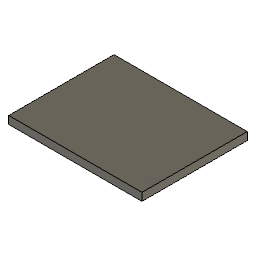
assembely (Autodesk Fusion 360 archive; units mm, degrees)
design "temp_sensor"
part number: 2025-12-15-20-50-01-731
Autodesk Fusion 360 part; units mm, degrees
sketch "Sketch1" plane through (0, 0, 0) normal (0, 0, 1) x (1, 0, 0)
  line L0 (0, 0) -> (25.3, 0)
  line L1 (25.3, 0) -> (25.3, 20)
  line L2 (25.3, 20) -> (0, 20)
  line L3 (0, 20) -> (0, 0)
  dimension "d1" = 25.3
  dimension "d2" = 20
  constraint horizontal L0
  constraint vertical L1
  constraint horizontal L2
  constraint vertical L3
  constraint coincident L0.start L3.end
  measures "d1" distance of L0.start L0.end
  measures "d2" distance of L0.start L2.end
extrude "Extrude1" add sketch "Sketch1" along normal blind 1.5

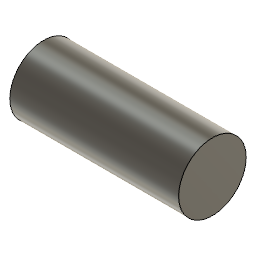
design "baterie"
part number: 2025-12-20-17-38-36-639
Autodesk Fusion 360 part; units mm, degrees
sketch "Sketch1" plane through (0, 0, 0) normal (1, 0, 0) x (0, 1, 0)
  circle A0 centre (0, 0) radius 13
  dimension "d1" = 26
  constraint coincident A0.centre origin
  measures "d1" diameter of A0
extrude "Extrude1" add sketch "Sketch1" along normal blind 65

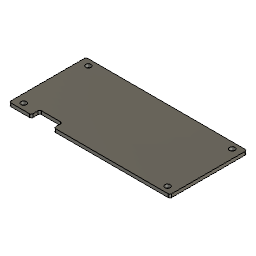
design "wood_back"
part number: 2025-12-15-21-34-38-126
Autodesk Fusion 360 part; units mm, degrees
sketch "Sketch1" plane through (0, 0, 0) normal (0, 0, 1) x (1, 0, 0)
  line L0 (0, 0) -> (96, 0)
  line L1 (96, 0) -> (96, 46)
  line L2 (96, 46) -> (0, 46)
  line L3 (0, 46) -> (0, 0)
  dimension "d1" = 96
  dimension "d2" = 46
  constraint horizontal L0
  constraint vertical L1
  constraint horizontal L2
  constraint vertical L3
  constraint coincident L0.start L3.end
  measures "d1" distance of L0.start L0.end
  measures "d2" distance of L0.start L2.end
extrude "Extrude1" add sketch "Sketch1" along normal blind 2
fillet "Fillet1" radius 1 4 edges at (96, 0, 1) (96, 46, 1) (0, 0, 1) (0, 46, 1)
sketch "Sketch2" plane through (0, 0, 2) normal (0, 0, 1) x (-1, 0, 0)
  arc A0 (-1, -46) -> (0, -45) centre (-1, -45) ccw
  line L0 (0, -45) -> (0, -1)
  arc A1 (0, -1) -> (-1, 0) centre (-1, -1) ccw
  line L1 (-1, 0) -> (-95, 0)
  arc A2 (-95, 0) -> (-96, -1) centre (-95, -1) ccw
  line L2 (-96, -1) -> (-96, -45)
  arc A3 (-96, -45) -> (-95, -46) centre (-95, -45) ccw
  line L3 (-95, -46) -> (-1, -46)
  line L4 (-13.3, 0) -> (-26.73, 0)
  line L5 (-26.73, 0) -> (-26.73, -4.065)
  line L6 (-25.73, -5.065) -> (-14.3, -5.065)
  line L7 (-13.3, -4.065) -> (-13.3, 0)
  arc A4 (-14.3, -5.065) -> (-13.3, -4.065) centre (-14.3, -4.065) ccw
  arc A5 (-26.73, -4.065) -> (-25.73, -5.065) centre (-25.73, -4.065) ccw
  point P0 (-13.3, -5.065)
  dimension "d7" = 13.43
  dimension "d8" = 5.065
  dimension "d9" = 13.3
  dimension "d10" = 5.065
  dimension "d11" = 1
  dimension "d12" = 1
  constraint horizontal L4
  constraint vertical L5
  constraint horizontal L6
  constraint vertical L7
  constraint coincident P0 L6
  constraint coincident P0 L7
  constraint tangent L6 A4
  constraint tangent L7 A4
  constraint tangent L5 A5
  constraint tangent L6 A5
  measures "d7" distance of L4.start L4.end
  measures "d8" distance of L4.start P0
  measures "d9" distance of L0 L7
  measures "d10" distance of L1 L6
  measures "d11" radius of A4
  measures "d12" radius of A5
extrude "Extrude2" cut sketch "Sketch2" against normal blind 2 contours L1 L4 L5 L6 L7 A4 A5
fillet "Fillet4" radius 1 2 edges at (13.3, 0, 1) (26.73, 0, 1)
sketch "Sketch5" plane through (0, 0, 2) normal (0, 0, 1) x (-1, 0, 0)
  arc A0 (-26.73, -1) -> (-27.73, 0) centre (-27.73, -1) ccw
  line L0 (-27.73, 0) -> (-95, 0)
  arc A1 (-95, 0) -> (-96, -1) centre (-95, -1) ccw
  line L1 (-96, -1) -> (-96, -45)
  arc A2 (-96, -45) -> (-95, -46) centre (-95, -45) ccw
  line L2 (-95, -46) -> (-1, -46)
  arc A3 (-1, -46) -> (0, -45) centre (-1, -45) ccw
  line L3 (0, -45) -> (0, -1)
  arc A4 (0, -1) -> (-1, 0) centre (-1, -1) ccw
  line L4 (-1, 0) -> (-12.3, 0)
  arc A5 (-12.3, 0) -> (-13.3, -1) centre (-12.3, -1) ccw
  line L5 (-13.3, -1) -> (-13.3, -4.065)
  arc A6 (-14.3, -5.065) -> (-13.3, -4.065) centre (-14.3, -4.065) ccw
  line L6 (-14.3, -5.065) -> (-25.73, -5.065)
  arc A7 (-26.73, -4.065) -> (-25.73, -5.065) centre (-25.73, -4.065) ccw
  line L7 (-26.73, -4.065) -> (-26.73, -1)
  circle A8 centre (-5.1, -3.75) radius 1.6
  circle A9 centre (-5.1, -42.25) radius 1.6
  circle A10 centre (-90.9, -3.75) radius 1.6
  circle A11 centre (-90.9, -42.25) radius 1.6
  dimension "d33" = 3.2
  dimension "d34" = 3.75
  dimension "d35" = 5.1
  dimension "d36" = 3.2
  dimension "d37" = 3.75
  dimension "d38" = 5.1
  dimension "d39" = 3.2
  dimension "d40" = 5.1
  dimension "d41" = 3.75
  dimension "d42" = 3.2
  dimension "d43" = 3.75
  dimension "d44" = 5.1
  measures "d33" diameter of A8
  measures "d34" distance of L4 A8.centre
  measures "d35" distance of L3 A8.centre
  measures "d36" diameter of A9
  measures "d37" distance of L2 A9.centre
  measures "d38" distance of L3 A9.centre
  measures "d39" diameter of A10
  measures "d40" distance of L1 A10.centre
  measures "d41" distance of L0 A10.centre
  measures "d42" diameter of A11
  measures "d43" distance of L2 A11.centre
  measures "d44" distance of L1 A11.centre
extrude "Extrude5" cut sketch "Sketch5" against normal blind 2 contours A8 | A9 | A10 | A11
equation "d8 = 4.69 mm - 0.375 mm + 0.75 mm"
equation "d10 = 4.69 mm - 0.375 mm + 0.75 mm"

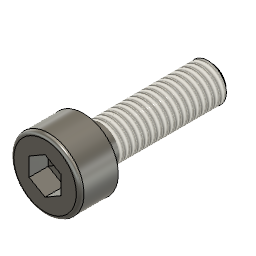
design "Broached Hexagon Socket Head Cap Screw ASME B18.3.1M - M3x0.5 x 10 Steel Grade 2 Plain"
description: Broached Hexagon Socket Head Cap Screw ASME B18.3.1M - M3x0.5 x 10
part number: BSHCS ASME B18.3.1M - M3x0.5 x 10 Steel Grade 2 Plain
Autodesk Fusion 360 part; units mm, degrees
sketch "Sketch1" plane through (0, 0, 0) normal (0, 1, 0) x (1, 0, 0)
  line L0 (-1.5, 0) -> (-1.5, 10)
  line L1 (-1.5, 10) -> (0, 10)
  line L2 (0, 10) -> (0, -3)
  line L3 (-1.5, 0) -> (-2.75, 0)
  line L4 (-2.75, 0) -> (-2.75, -3)
  line L5 (-2.75, -3) -> (0, -3)
  dimension "d101" = 10
  dimension "d102" = 3
  dimension "d109" = 5.5
  dimension "d110" = 3
  constraint perpendicular L0 L1
  constraint collinear origin L1.end L2.end
  constraint perpendicular L0 L3
  constraint coincident origin L3
  constraint vertical L2
  constraint coincident L2 L5.end
  constraint perpendicular L2 L5
  measures "d101" distance of origin L1
  measures "d102" distance of L3.end L5
revolve "Revolve1" add sketch "Sketch1" angle 360 about axis through (0, 0, -10) along (0, 0, 1)
ref_plane "WorkPlane1" through (0, 0, 3) normal (0, 0, 1) x (1, 0, 0)
sketch "Sketch6" plane through (0, 0, 3) normal (0, 0, 1) x (1, 0, 0)
  line L0 (0, -1.4434) -> (1.25, -0.7217)
  line L1 (1.25, -0.7217) -> (1.25, 0.7217)
  line L2 (1.25, 0.7217) -> (0, 1.4434)
  line L3 (0, 1.4434) -> (-1.25, 0.7217)
  line L4 (-1.25, 0.7217) -> (-1.25, -0.7217)
  line L5 (-1.25, -0.7217) -> (0, -1.4434)
  dimension "d111" = 2.5
  constraint vertical L1
  measures "d111" distance of L1 L4
extrude "Extrude1" cut sketch "Sketch6" against normal blind 1.5
extrude "Extrude2" cut 1 faces at (0.4167, -0.2406, 1.5) along direction (0, 0, -1) blind 1.5 draft -85
thread "Thread3" "ANSI Metric M Profile 3.0 M3x0.5 M3x0.5 4g6g" major diameter 2.927 minor diameter 2.369 pitch 0.5 angle 60 resizes the face on face at (-1.4925, 0.1494, -6.6667) from (0, 0, -1.3067) to (0, 0, -10)
fillet "Fillet4" radius 0.3 1 edges at (-2.5639, 0.9944, 3)
sketch "Sketch7" plane through (0, 0, 0) normal (0, 1, 0) x (1, 0, 0)
  line L0 (-1.53, 10) -> (-1.53, 9.6933)
  line L1 (-1.53, 9.6933) -> (-1.1933, 10)
  line L2 (0, 10) -> (0, -3)
  line L3 (-1.53, 10) -> (0, 10)
  dimension "d104" = 1.1933
  dimension "d105" = 1.53
  dimension "d106" = 0.3067
  constraint coincident L2.start L3.end
  constraint perpendicular L2 L3
  constraint coincident L1.end L3
  constraint perpendicular L0 L3
  measures "d104" distance of L1.end L2
  measures "d105" distance of L0 L2.start
  measures "d106" distance of L0.end L3
revolve "Revolve3" cut sketch "Sketch7" angle 360 about axis through (0, 0, 1.75) along (0, 0, 1)
equation "adsk_nomlen = 10.00 mm"
equation "adsk_headh = 3.00 mm"
equation "adsk_headdia = 5.50 mm"
equation "adsk_nomdia = 3.00 mm"
equation "adsk_philwidth = 2.50 mm"
equation "d31 = -adsk_phildepth"
equation "adsk_phildepth = 1.50 mm"
equation "d71 = adsk_headh"
equation "d76 = -adsk_phildepth"
equation "adsk_thrlen = 8.693275 mm"
equation "d86 = adsk_nomdia * 0.1"
equation "adsk_startlen = 0.306725 mm"
equation "adsk_endpointdia = 2.38655 mm"
equation "d101 = adsk_nomlen"
equation "d102 = adsk_headh"
equation "d104 = adsk_endpointdia / 2"
equation "d105 = adsk_nomdia * 0.51"
equation "d106 = adsk_startlen"
equation "d108 = min(adsk_thrlen; adsk_nomlen - 0.001 mm)"
equation "d109 = adsk_headdia"
equation "d110 = adsk_nomdia"
equation "d111 = adsk_philwidth"

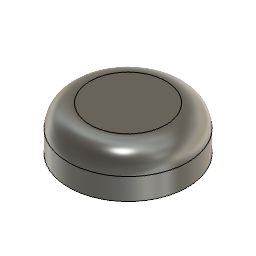
design "gumova_nozicka"
part number: 2025-12-22-20-39-36-986
Autodesk Fusion 360 part; units mm, degrees
sketch "Sketch1" plane through (0, 0, 0) normal (0, 0, 1) x (1, 0, 0)
  circle A0 centre (0, 0) radius 5.5
  dimension "d1" = 11
  constraint coincident A0.centre origin
  measures "d1" diameter of A0
extrude "Extrude1" add sketch "Sketch1" along normal blind 4
fillet "Fillet1" radius 2 1 edges at (-5.1278, -1.9889, 4)

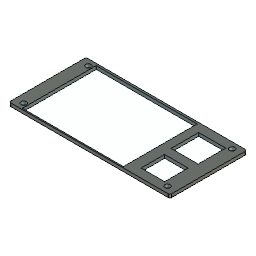
design "wood_front"
part number: 2025-12-15-21-06-19-821
Autodesk Fusion 360 part; units mm, degrees
sketch "Sketch1" plane through (0, 0, 0) normal (0, 0, 1) x (1, 0, 0)
  line L0 (0, 0) -> (96, 0)
  line L1 (96, 0) -> (96, 46)
  line L2 (96, 46) -> (0, 46)
  line L3 (0, 46) -> (0, 0)
  dimension "d1" = 96
  dimension "d2" = 46
  constraint horizontal L0
  constraint vertical L1
  constraint horizontal L2
  constraint vertical L3
  measures "d1" distance of L0.start L0.end
  measures "d2" distance of L0.start L2.end
extrude "Extrude1" add sketch "Sketch1" along normal blind 2
fillet "Fillet1" radius 1 4 edges at (96, 0, 1) (96, 46, 1) (0, 46, 1) (0, 0, 1)
sketch "Sketch2" plane through (0, 0, 2) normal (0, 0, 1) x (-1, 0, 0)
  arc A0 (0, -1) -> (-1, 0) centre (-1, -1) ccw
  line L0 (-1, 0) -> (-95, 0)
  arc A1 (-95, 0) -> (-96, -1) centre (-95, -1) ccw
  line L1 (-96, -1) -> (-96, -45)
  arc A2 (-96, -45) -> (-95, -46) centre (-95, -45) ccw
  line L2 (-95, -46) -> (-1, -46)
  arc A3 (-1, -46) -> (0, -45) centre (-1, -45) ccw
  line L3 (0, -45) -> (0, -1)
  circle A4 centre (-5.1, -42.25) radius 1.6
  circle A5 centre (-90.9, -42.25) radius 1.6
  circle A6 centre (-90.9, -3.75) radius 1.6
  circle A7 centre (-5.1, -3.75) radius 1.6
  dimension "d7" = 3.2
  dimension "d8" = 3.75
  dimension "d9" = 5.1
  dimension "d10" = 3.2
  dimension "d11" = 3.2
  dimension "d12" = 3.2
  dimension "d13" = 3.75
  dimension "d14" = 5.1
  dimension "d15" = 3.75
  dimension "d16" = 5.1
  dimension "d17" = 5.1
  dimension "d18" = 3.75
  measures "d7" diameter of A4
  measures "d8" distance of L2 A4.centre
  measures "d9" distance of L3 A4.centre
  measures "d10" diameter of A5
  measures "d11" diameter of A6
  measures "d12" diameter of A7
  measures "d13" distance of L0 A7.centre
  measures "d14" distance of L3 A7.centre
  measures "d15" distance of L0 A6.centre
  measures "d16" distance of L1 A6.centre
  measures "d17" distance of L1 A5.centre
  measures "d18" distance of L2 A5.centre
extrude "Extrude2" cut sketch "Sketch2" against normal blind 2 contours A4 | A5 | A6 | A7
sketch "Sketch3" plane through (0, 0, 2) normal (0, 0, 1) x (-1, 0, 0)
  circle A0 centre (-90.9, -3.75) radius 1.6
  circle A1 centre (-5.1, -3.75) radius 1.6
  circle A2 centre (-90.9, -42.25) radius 1.6
  circle A3 centre (-5.1, -42.25) radius 1.6
  arc A4 (0, -1) -> (-1, 0) centre (-1, -1) ccw
  line L0 (-1, 0) -> (-95, 0)
  arc A5 (-95, 0) -> (-96, -1) centre (-95, -1) ccw
  line L1 (-96, -1) -> (-96, -45)
  arc A6 (-96, -45) -> (-95, -46) centre (-95, -45) ccw
  line L2 (-95, -46) -> (-1, -46)
  arc A7 (-1, -46) -> (0, -45) centre (-1, -45) ccw
  line L3 (0, -45) -> (0, -1)
  line L4 (-2.5, -46) -> (-2.5, 0) construction
  line L5 (-7.3, -46) -> (-7.3, 0)
  line L6 (-93.5, -46) -> (-93.5, 0)
  line L7 (-88.5, -46) -> (-88.5, 0)
  line L8 (-7.3, -44.75) -> (-67.5, -44.75)
  line L9 (-67.5, -44.75) -> (-67.5, -0.75)
  line L10 (-67.5, -0.75) -> (-7.3, -0.75)
  line L11 (-7.3, -0.75) -> (-7.3, -44.75)
  line L12 (0, -23) -> (-96, -23) construction
  dimension "d21" = 2.6
  dimension "d22" = 4.8
  dimension "d23" = 2.6
  dimension "d24" = 5
  dimension "d26" = 44
  dimension "d27" = 44
  dimension "d29" = 21.75
  dimension "d30" = 22
  dimension "d31" = 4.8
  dimension "d32" = 21
  dimension "d34" = 60.2
  constraint coincident L2 L4.start
  constraint perpendicular L2 L4
  constraint coincident L0 L4.end
  constraint coincident L2 L5.start
  constraint perpendicular L2 L5
  constraint coincident L0 L5.end
  constraint coincident L2 L6.start
  constraint coincident L0 L6.end
  constraint coincident L2 L7.start
  constraint coincident L0 L7.end
  constraint perpendicular L0 L7
  constraint horizontal L8
  constraint vertical L9
  constraint horizontal L10
  constraint vertical L11
  constraint coincident L3 L12.start
  constraint coincident L1 L12.end
  constraint perpendicular L1 L12
  measures "d21" distance of A3.centre L4
  measures "d22" distance of L4 L5
  measures "d23" distance of A0.centre L6
  measures "d24" distance of L6 L7
  measures "d26" distance of L8.start L10.end
  measures "d27" distance of A5.end L1.end
  measures "d29" distance of L8 L12
  measures "d30" distance of A7.end L12
  measures "d31" distance of L4 L11
  measures "d32" distance of L7 L9
  measures "d34" distance of L5 L9
extrude "Extrude3" cut sketch "Sketch3" against normal blind 2 contours L5 L8 L9 L10 L11
sketch "Sketch4" plane through (0, 0, 2) normal (0, 0, 1) x (-1, 0, 0)
  line L0 (-67.5, -44.75) -> (-67.5, -0.75)
  line L1 (-67.5, -0.75) -> (-7.3, -0.75)
  line L2 (-7.3, -0.75) -> (-7.3, -44.75)
  line L3 (-7.3, -44.75) -> (-67.5, -44.75)
  circle A0 centre (-90.9, -3.75) radius 1.6
  circle A1 centre (-5.1, -3.75) radius 1.6
  circle A2 centre (-90.9, -42.25) radius 1.6
  circle A3 centre (-5.1, -42.25) radius 1.6
  arc A4 (0, -1) -> (-1, 0) centre (-1, -1) ccw
  line L4 (-1, 0) -> (-95, 0)
  arc A5 (-95, 0) -> (-96, -1) centre (-95, -1) ccw
  line L5 (-96, -1) -> (-96, -45)
  arc A6 (-96, -45) -> (-95, -46) centre (-95, -45) ccw
  line L6 (-95, -46) -> (-1, -46)
  arc A7 (-1, -46) -> (0, -45) centre (-1, -45) ccw
  line L7 (0, -45) -> (0, -1)
  line L8 (-93.5, -46) -> (-93.5, 0)
  line L9 (-88.5, -46) -> (-88.5, 0)
  line L10 (-73.4, -39.75) -> (-87.8, -39.75)
  line L11 (-87.8, -39.75) -> (-87.8, -25.35)
  line L12 (-87.8, -25.35) -> (-73.4, -25.35)
  line L13 (-73.4, -25.35) -> (-73.4, -39.75)
  line L14 (-74.6, -18.25) -> (-86.6, -18.25)
  line L15 (-86.6, -18.25) -> (-86.6, -6.25)
  line L16 (-86.6, -6.25) -> (-74.6, -6.25)
  line L17 (-74.6, -6.25) -> (-74.6, -18.25)
  line L18 (-72.4, -40.75) -> (-88.8, -40.75)
  line L19 (-88.8, -40.75) -> (-88.8, -24.35)
  line L20 (-88.8, -24.35) -> (-72.4, -24.35)
  line L21 (-72.4, -24.35) -> (-72.4, -40.75)
  line L22 (-73.6, -5.25) -> (-73.6, -19.25)
  line L23 (-73.6, -19.25) -> (-87.6, -19.25)
  line L24 (-87.6, -19.25) -> (-87.6, -5.25)
  line L25 (-87.6, -5.25) -> (-73.6, -5.25)
  dimension "d38" = 2.6
  dimension "d39" = 5
  dimension "d40" = 14.4
  dimension "d41" = 14.4
  dimension "d42" = 5.7
  dimension "d44" = 12
  dimension "d45" = 12
  dimension "d46" = 6.9
  dimension "d47" = 7.1
  dimension "d48" = -1
  dimension "d49" = -1
  dimension "d50" = 5
  constraint coincident L6 L8.start
  constraint coincident L4 L8.end
  constraint perpendicular L4 L8
  constraint coincident L6 L9.start
  constraint coincident L4 L9.end
  constraint perpendicular L4 L9
  constraint horizontal L10
  constraint vertical L11
  constraint horizontal L12
  constraint vertical L13
  constraint horizontal L14
  constraint vertical L15
  constraint horizontal L16
  constraint vertical L17
  measures "d38" distance of A2.centre L8
  measures "d39" distance of L8 L9
  measures "d40" distance of L10.start L10.end
  measures "d41" distance of L10.start L12.end
  measures "d42" distance of L8 L11
  measures "d44" distance of L14.start L14.end
  measures "d45" distance of L14.start L16.end
  measures "d46" distance of L8 L15
  measures "d47" distance of L12 L14
  measures "d50" distance of L3 L10
extrude "Extrude4" cut sketch "Sketch4" against normal blind 2 contours L9 L18 L20 L21 | L10 L11 L12 L13 | L14 L15 L16 L17 | L22 L23 L24 L25
sketch "Sketch5" plane through (0, 0, 2) normal (0, 0, 1) x (-1, 0, 0)
  line L0 (-88.5, -40.75) -> (-88.5, -24.35)
  line L1 (-88.5, -24.35) -> (-72.4, -24.35)
  line L2 (-72.4, -24.35) -> (-72.4, -40.75)
  line L3 (-72.4, -40.75) -> (-88.5, -40.75)
  line L4 (-73.6, -19.25) -> (-87.6, -19.25)
  line L5 (-87.6, -19.25) -> (-87.6, -5.25)
  line L6 (-87.6, -5.25) -> (-73.6, -5.25)
  line L7 (-73.6, -5.25) -> (-73.6, -19.25)
  line L8 (-67.5, -44.75) -> (-67.5, -0.75)
  line L9 (-67.5, -0.75) -> (-7.3, -0.75)
  line L10 (-7.3, -0.75) -> (-7.3, -44.75)
  line L11 (-7.3, -44.75) -> (-67.5, -44.75)
  circle A0 centre (-90.9, -3.75) radius 1.6
  circle A1 centre (-5.1, -3.75) radius 1.6
  circle A2 centre (-90.9, -42.25) radius 1.6
  circle A3 centre (-5.1, -42.25) radius 1.6
  arc A4 (0, -1) -> (-1, 0) centre (-1, -1) ccw
  line L12 (-1, 0) -> (-95, 0)
  arc A5 (-95, 0) -> (-96, -1) centre (-95, -1) ccw
  line L13 (-96, -1) -> (-96, -45)
  arc A6 (-96, -45) -> (-95, -46) centre (-95, -45) ccw
  line L14 (-95, -46) -> (-1, -46)
  arc A7 (-1, -46) -> (0, -45) centre (-1, -45) ccw
  line L15 (0, -45) -> (0, -1)
  dimension "d53" = 3.75
  dimension "d54" = 3.75
  dimension "d55" = 3.75
  measures "d53" distance of A1.centre L12
  measures "d54" distance of A2.centre L14
  measures "d55" distance of A0.centre L12
equation "d21 = 1 mm + ( ( 3.2 / 2 ) * 1 mm )"
equation "d29 = ( 43.5 / 2 ) * 1 mm"
equation "d38 = ( 3.2 / 2 ) * 1 mm + 1 mm"

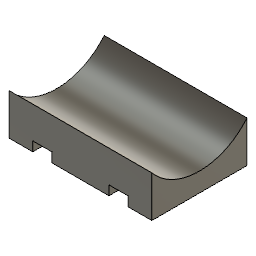
design "battery_hold"
part number: 2025-12-20-17-48-02-593
Autodesk Fusion 360 part; units mm, degrees
sketch "Sketch1" plane through (0, 0, 0) normal (0, 0, 1) x (1, 0, 0)
sketch "Sketch2" plane through (0, 0, 0) normal (0, 0, 1) x (1, 0, 0)
  line L0 (0, 0) -> (30, 0)
  line L1 (30, 0) -> (30, 20)
  line L2 (30, 20) -> (0, 20)
  line L3 (0, 20) -> (0, 0)
  dimension "d1" = 30
  dimension "d2" = 20
  constraint horizontal L0
  constraint vertical L1
  constraint horizontal L2
  constraint vertical L3
  constraint coincident L0.start L3.end
  measures "d1" distance of L0.start L0.end
  measures "d2" distance of L0.start L2.end
extrude "Extrude1" add sketch "Sketch2" along normal blind 15
sketch "Sketch3" plane through (30, 0, 0) normal (1, 0, 0) x (0, 1, 0)
  line L0 (0, 0) -> (20, 0)
  line L1 (20, 0) -> (20, 15)
  line L2 (20, 15) -> (0, 15)
  line L3 (0, 15) -> (0, 0)
  circle A0 centre (10, 17) radius 13
  dimension "d5" = 26
  dimension "d6" = 17
  dimension "d7" = 10
  measures "d5" diameter of A0
  measures "d6" distance of L0 A0.centre
  measures "d7" distance of L3 A0.centre
extrude "Extrude2" cut sketch "Sketch3" against normal blind 60 contours L1 L2 L3 A0 | L1 L2 L3 A0
sketch "Sketch4" plane through (0, 0, 0) normal (0, -1, 0) x (1, 0, 0)
  line L0 (30, 8.6934) -> (0, 8.6934)
  line L1 (0, 8.6934) -> (0, 0)
  line L2 (0, 0) -> (30, 0)
  line L3 (30, 0) -> (30, 8.6934)
  line L4 (5, 0) -> (9, 0)
  line L5 (9, 0) -> (9, 2)
  line L6 (9, 2) -> (5, 2)
  line L7 (5, 2) -> (5, 0)
  line L8 (21, 0) -> (25, 0)
  line L9 (25, 0) -> (25, 2)
  line L10 (25, 2) -> (21, 2)
  line L11 (21, 2) -> (21, 0)
  dimension "d10" = 4
  dimension "d11" = 2
  dimension "d12" = 4
  dimension "d13" = 2
  dimension "d14" = 5
  dimension "d15" = 5
  constraint horizontal L4
  constraint vertical L5
  constraint horizontal L6
  constraint vertical L7
  constraint coincident L2 L4.start
  constraint horizontal L8
  constraint vertical L9
  constraint horizontal L10
  constraint vertical L11
  constraint coincident L2 L8.start
  measures "d10" distance of L4.start L4.end
  measures "d11" distance of L4.start L6.end
  measures "d12" distance of L8.start L8.end
  measures "d13" distance of L8.start L10.end
  measures "d14" distance of L3 L9
  measures "d15" distance of L1 L7
extrude "Extrude3" cut sketch "Sketch4" against normal blind 50 contours L2 L8 L9 L10 L11 | L2 L4 L5 L6 L7

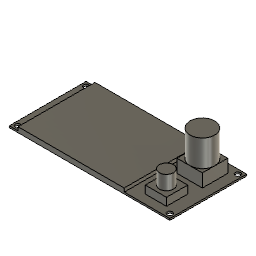
design "display"
part number: 2025-12-15-16-48-16-631
Autodesk Fusion 360 part; units mm, degrees
sketch "Sketch1" plane through (0, 0, 0) normal (0, 0, 1) x (1, 0, 0)
  line L0 (0, 0) -> (90.8, 0)
  line L1 (90.8, 0) -> (90.8, 43.5)
  line L2 (90.8, 43.5) -> (0, 43.5)
  line L3 (0, 43.5) -> (0, 0)
  line L4 (5, 0) -> (65, 0)
  line L5 (65, 0) -> (65, 43.5)
  line L6 (65, 43.5) -> (5, 43.5)
  line L7 (5, 43.5) -> (5, 0)
  circle A0 centre (2.5, 2.5) radius 1.5
  circle A1 centre (2.5, 41) radius 1.5
  dimension "d1" = 90.8
  dimension "d2" = 43.5
  dimension "d3" = 60
  dimension "d4" = 65
  dimension "d5" = 3
  dimension "d6" = 2.5
  dimension "d7" = 2.5
  dimension "d8" = 3
  dimension "d9" = 2.5
  dimension "d10" = 2.5
  constraint horizontal L0
  constraint vertical L1
  constraint horizontal L2
  constraint vertical L3
  constraint coincident L0.start L3.end
  constraint horizontal L4
  constraint vertical L5
  constraint horizontal L6
  constraint vertical L7
  constraint coincident L2 L5.end
  constraint coincident L0 L4.start
  measures "d1" distance of L0.start L0.end
  measures "d2" distance of L0.start L2.end
  measures "d3" distance of L5 L7
  measures "d4" distance of L3 L5
  measures "d5" diameter of A0
  measures "d6" distance of L0 A0.centre
  measures "d7" distance of L3 A0.centre
  measures "d8" diameter of A1
  measures "d9" distance of L2 A1.centre
  measures "d10" distance of L3 A1.centre
extrude "Extrude1" add sketch "Sketch1" along normal blind 1
sketch "Sketch2" plane through (0, 0, 1) normal (0, 0, 1) x (-1, 0, 0)
  circle A0 centre (-2.5, -2.5) radius 1.5
  circle A1 centre (-2.5, -41) radius 1.5
  line L0 (-90.8, -43.5) -> (0, -43.5)
  line L1 (0, -43.5) -> (0, 0)
  line L2 (0, 0) -> (-90.8, 0)
  line L3 (-90.8, 0) -> (-90.8, -43.5)
  line L4 (-5, 0) -> (-65, 0)
  line L5 (-65, 0) -> (-65, -43.5)
  line L6 (-65, -43.5) -> (-5, -43.5)
  line L7 (-5, -43.5) -> (-5, 0)
  dimension "d13" = 60
  dimension "d14" = 65
  constraint horizontal L4
  constraint vertical L5
  constraint horizontal L6
  constraint vertical L7
  constraint coincident L0 L5.end
  constraint coincident L2 L4.start
  measures "d13" distance of L5 L7
  measures "d14" distance of L1 L5
extrude "Extrude2" add sketch "Sketch2" along normal blind 1 contours L0 L2 L4 L5 L6 L7
sketch "Sketch3" plane through (0, 0, 1) normal (0, 0, 1) x (-1, 0, 0)
  line L0 (-65, -43.5) -> (-65, 0)
  line L1 (-65, 0) -> (-90.8, 0)
  line L2 (-90.8, 0) -> (-90.8, -43.5)
  line L3 (-90.8, -43.5) -> (-65, -43.5)
  line L4 (-83.9, -5) -> (-71.9, -5)
  line L5 (-71.9, -5) -> (-71.9, -17)
  line L6 (-71.9, -17) -> (-83.9, -17)
  line L7 (-83.9, -17) -> (-83.9, -5)
  line L8 (-77.9, -43.5) -> (-77.9, 0) construction
  line L9 (-70.7, -38.5) -> (-85.1, -38.5)
  line L10 (-85.1, -38.5) -> (-85.1, -24.1)
  line L11 (-85.1, -24.1) -> (-70.7, -24.1)
  line L12 (-70.7, -24.1) -> (-70.7, -38.5)
  dimension "d17" = 12
  dimension "d18" = 12
  dimension "d19" = 12.9
  dimension "d20" = 6
  dimension "d21" = 5
  dimension "d22" = 14.4
  dimension "d23" = 14.4
  dimension "d24" = 5
  dimension "d25" = 7.2
  constraint horizontal L4
  constraint vertical L5
  constraint horizontal L6
  constraint vertical L7
  constraint coincident L3 L8.start
  constraint coincident L1 L8.end
  constraint perpendicular L1 L8
  constraint horizontal L9
  constraint vertical L10
  constraint horizontal L11
  constraint vertical L12
  measures "d17" distance of L4.start L4.end
  measures "d18" distance of L4.start L6.end
  measures "d19" distance of L2 L8
  measures "d20" distance of L5 L8
  measures "d21" distance of L1 L4
  measures "d22" distance of L9.start L9.end
  measures "d23" distance of L9.start L11.end
  measures "d24" distance of L3 L9
  measures "d25" distance of L8 L10
extrude "Extrude3" add sketch "Sketch3" along normal blind 12.4 contours L4 L5 L6 L7 | L9 L10 L11 L12
extrude "Extrude4" add 1 faces at (80.3, 33.7, 13.4) along direction (0, 0, 1) blind 10
sketch "Sketch4" plane through (0, 0, 13.4) normal (0, 0, 1) x (-1, 0, 0)
  line L0 (-83.9, -17) -> (-71.9, -17)
  line L1 (-71.9, -17) -> (-71.9, -5)
  line L2 (-71.9, -5) -> (-83.9, -5)
  line L3 (-83.9, -5) -> (-83.9, -17)
  circle A0 centre (-77.9, -11) radius 4
  dimension "d30" = 8
  dimension "d31" = 6
  dimension "d32" = 6
  measures "d30" diameter of A0
  measures "d31" distance of L0 A0.centre
  measures "d32" distance of L1 A0.centre
extrude "Extrude5" cut sketch "Sketch4" against normal blind 8
extrude "Extrude6" add 1 faces at (45, 14.5, 2) along direction (0, 0, 1) blind 1
sketch "Sketch5" plane through (0, 0, 1) normal (0, 0, 1) x (-1, 0, 0)
  line L0 (-70.7, -24.1) -> (-70.7, -38.5)
  line L1 (-70.7, -38.5) -> (-85.1, -38.5)
  line L2 (-85.1, -38.5) -> (-85.1, -24.1)
  line L3 (-85.1, -24.1) -> (-70.7, -24.1)
  line L4 (-83.9, -17) -> (-83.9, -5)
  line L5 (-83.9, -5) -> (-71.9, -5)
  line L6 (-71.9, -5) -> (-71.9, -17)
  line L7 (-71.9, -17) -> (-83.9, -17)
  line L8 (-65, -43.5) -> (-65, 0)
  line L9 (-65, 0) -> (-90.8, 0)
  line L10 (-90.8, 0) -> (-90.8, -43.5)
  line L11 (-90.8, -43.5) -> (-65, -43.5)
  circle A0 centre (-88.3, -2.5) radius 1.5
  circle A1 centre (-88.3, -41) radius 1.5
  dimension "d37" = 3
  dimension "d38" = 2.5
  dimension "d39" = 2.5
  dimension "d40" = 3
  dimension "d41" = 2.5
  dimension "d42" = 2.5
  measures "d37" diameter of A0
  measures "d38" distance of L10 A0.centre
  measures "d39" distance of L9 A0.centre
  measures "d40" diameter of A1
  measures "d41" distance of L11 A1.centre
  measures "d42" distance of L10 A1.centre
extrude "Extrude7" cut sketch "Sketch5" against normal blind 1 contours A0 | A1
extrude "Extrude8" cut 1 faces at (80.3, 33.7, 23.4) along direction (0, 0, -1) blind 15
sketch "Sketch6" plane through (0, 0, 8.4) normal (0, 0, 1) x (-1, 0, 0)
  line L0 (-70.7, -24.1) -> (-85.1, -24.1)
  line L1 (-85.1, -24.1) -> (-85.1, -38.5)
  line L2 (-85.1, -38.5) -> (-70.7, -38.5)
  line L3 (-70.7, -38.5) -> (-70.7, -24.1)
  circle A0 centre (-78.1, -31.1) radius 7
  dimension "d47" = 14
  dimension "d48" = 7
  dimension "d49" = 7
  measures "d47" diameter of A0
  measures "d48" distance of L0 A0.centre
  measures "d49" distance of L1 A0.centre
extrude "Extrude9" add sketch "Sketch6" along normal blind 15 contours A0
equation "d25 = ( 14.4 / 2 ) * 1 mm"
